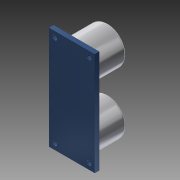
# Autodesk Inventor part: HC-SR04 Sonar
Saved by Autodesk Inventor 2015 (Build 190159000, 159)
## iProperties
Created: 2015-11-02
Part Number: HC-SR04 Sonar
Material: Generic
Document SubType Name: Modeling
Designer: James
Density: 1 g/cm^3
Appearance: Default
Author: James
Autodesk Inventor part; units mm, degrees
ref_plane "YZ Plane" through (0, 0, 0) normal (1, 0, 0) x (0, 1, 0)
ref_plane "XZ Plane" through (0, 0, 0) normal (0, 1, 0) x (-1, 0, 0)
ref_plane "XY Plane" through (0, 0, 0) normal (0, 0, 1) x (1, 0, 0)
sketch "Sketch1" plane through (0, 0, 0) normal (0, 1, 0) x (-1, 0, 0)
  line L0 (-10, 22.5) -> (-10, -22.5)
  line L1 (-10, -22.5) -> (10, -22.5)
  line L2 (10, -22.5) -> (10, 22.5)
  line L3 (10, 22.5) -> (-10, 22.5)
  line L4 (-10, 22.5) -> (10, -22.5) construction
  line L5 (-10, -22.5) -> (10, 22.5) construction
  point P0 (0, 0)
  dimension "d0" = 45
  dimension "d1" = 20
  constraints: 12 end point, 2 midpoint, 2 parallel, 1 perpendicular, 1 vertical
  measures "d0" distance of L0.start L0.end
  measures "d1" distance of L1.end L0.end
extrude "Extrusion1" add sketch "Sketch1" along normal blind 2
sketch "Sketch2" plane through (0, 2, 0) normal (0, 1, 0) x (1, 0, 0)
  line L0 (7.5, -20) -> (7.5, 20)
  line L1 (7.5, 20) -> (-7.5, 20)
  line L2 (-7.5, 20) -> (-7.5, -20)
  line L3 (-7.5, -20) -> (7.5, -20)
  line L4 (7.5, -20) -> (-7.5, 20) construction
  line L5 (7.5, 20) -> (-7.5, -20) construction
  circle A0 centre (-7.5, -20) radius 1
  circle A1 centre (7.5, -20) radius 1
  circle A2 centre (7.5, 20) radius 1
  circle A3 centre (-7.5, 20) radius 1
  point P0 (0, 0)
  dimension "d25" = 40
  dimension "d26" = 15
  dimension "d27" = 2
  dimension "d28" = 2
  dimension "d29" = 2
  dimension "d30" = 2
  constraints: 12 end point, 4 centre point, 4 coincident, 2 midpoint, 2 parallel, 1 perpendicular, 1 vertical
  measures "d25" distance of L0.start L0.end
  measures "d26" distance of L1.end L0.end
  measures "d27" diameter of A0
  measures "d28" diameter of A1
  measures "d29" diameter of A2
  measures "d30" diameter of A3
extrude "Extrusion2" cut sketch "Sketch2" against normal blind 2 contours L3 A1 L0 | L0 A1 L3 | A2 L1 L0 | L0 L1 A2 | A0 L2 L3 | L3 L2 A0 | A3 L2 L1 | L1 L2 A3
sketch "Sketch3" plane through (0, 2, 0) normal (0, 1, 0) x (1, 0, 0)
  circle A0 centre (0, -13.5) radius 8
  circle A1 centre (0, 13.5) radius 8
  dimension "d33" = 16
  dimension "d34" = 16
  constraints: 2 centre point
  measures "d33" diameter of A0
  measures "d34" diameter of A1
extrude "Extrusion3" add sketch "Sketch3" along normal blind 13.8
fillet "Fillet1" radius 1 2 edges at (-8, 15.8, -13.5) (-8, 15.8, 13.5)
sketch "Sketch4" plane through (0, 15.8, 13.5) normal (0, 1, 0) x (1, 0, 0)
  circle A0 centre (0, 0) radius 8 projected
  circle A1 centre (0, 27) radius 8 projected
  circle A2 centre (0, 0) radius 6.5
  circle A3 centre (0, 27) radius 6.5
  dimension "d35" = 13
  dimension "d36" = 13
  constraints: 2 centre point, 2 coincident
  measures "d35" diameter of A2
  measures "d36" diameter of A3
extrude "Extrusion4" cut sketch "Sketch4" against normal blind 1 contours A2 | A3
body "Solid1"
